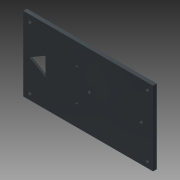
# Autodesk Inventor part: Front back
Saved by Autodesk Inventor 2015 (Build 190159000, 159)
## iProperties
Created: 2015-09-07
Part Number: Front back
Material: Iron, Gray
Document SubType Name: Modeling
Designer: Silas
Density: 7.15 g/cm^3
Appearance: Iron Gray
Mass: 131.393 g
Surface Area: 135.709 cm^2
Volume: 18.3766 cm^3
Author: Silas
Autodesk Inventor part; units mm, degrees
ref_plane "YZ Plane" through (0, 0, 0) normal (1, 0, 0) x (0, 1, 0)
ref_plane "XZ Plane" through (0, 0, 0) normal (0, 1, 0) x (-1, 0, 0)
ref_plane "XY Plane" through (0, 0, 0) normal (0, 0, 1) x (1, 0, 0)
sketch "Sketch1" plane through (0, 0, 0) normal (0, 1, 0) x (-1, 0, 0)
  line L0 (52.5, 30) -> (-52.5, 30)
  line L1 (-52.5, 30) -> (-52.5, -30)
  line L2 (-52.5, -30) -> (52.5, -30)
  line L3 (52.5, -30) -> (52.5, 30)
  line L4 (52.5, 0) -> (-52.5, 0) construction
  circle A0 centre (-42.5, 0) radius 1.5
  circle A1 centre (-0.5, 0) radius 1.5
  line L5 (-47.5, 25) -> (47.5, 25) construction
  line L6 (47.5, 25) -> (47.5, -25) construction
  line L7 (47.5, -25) -> (-47.5, -25) construction
  line L8 (-47.5, -25) -> (-47.5, 25) construction
  circle A2 centre (47.5, 25) radius 1.5
  circle A3 centre (47.5, -25) radius 1.5
  circle A4 centre (-47.5, 25) radius 1.5
  circle A5 centre (-47.5, -25) radius 1.5
  line L9 (47.5, 0) -> (34.5096, -7.5)
  line L10 (34.5096, -7.5) -> (34.5096, 7.5)
  line L11 (34.5096, 7.5) -> (47.5, 0)
  circle A6 centre (9.5, -13) radius 1
  circle A7 centre (9.5, 13) radius 1
  line L12 (9.5, -30) -> (9.5, 30) construction
  point P0 (0, 0)
  point P1 (0, 0)
  point P2 (38.8397, 0)
  dimension "d0" = 105
  dimension "d1" = 60
  dimension "d2" = 3
  dimension "d3" = 3
  dimension "d4" = 42
  dimension "d5" = 5
  dimension "d6" = 3
  dimension "d7" = 3
  dimension "d8" = 3
  dimension "d9" = 3
  dimension "d10" = 15
  dimension "d11" = 10
  dimension "d17" = 2
  dimension "d18" = 2
  dimension "d19" = 26
  dimension "d20" = 10
  constraints: 26 end point, 8 centre point, 8 point on line, 5 coincident, 4 midpoint, 4 parallel, 3 perpendicular, 1 horizontal, 1 symmetric about line, 10 other
  measures "d0" distance of L0.start L0.end
  measures "d1" distance of L2.end L0.start
  measures "d2" diameter of A0
  measures "d3" diameter of A1
  measures "d4" distance of A1.centre A0.centre
  measures "d5" distance between parallel lines of L0 L5
  measures "d6" diameter of A2
  measures "d7" diameter of A3
  measures "d8" diameter of A4
  measures "d9" diameter of A5
  measures "d10" distance of L9.end L10.end
  measures "d11" distance from line of L1 A0.centre
  measures "d17" diameter of A6
  measures "d18" diameter of A7
  measures "d19" distance of A7.centre A6.centre
  measures "d20" distance from line of L12 A1.centre
extrude "Extrusion1" add sketch "Sketch1" along normal blind 3
chamfer "Chamfer1" distance 2 angle 45 3 edges at (-41.0048, 3, -3.75) (-41.0048, 3, 3.75) (-34.5096, 3, 0)
body "Solid1"
